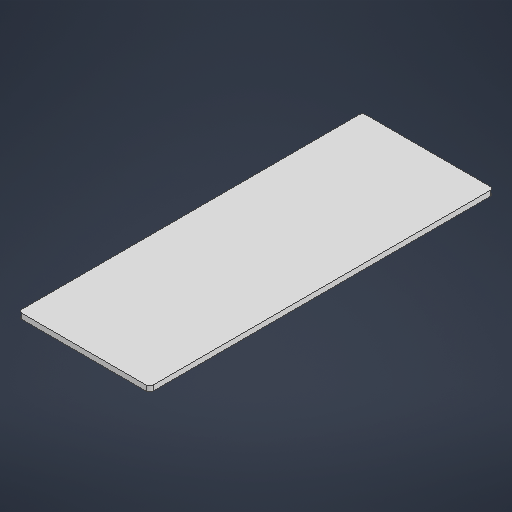
# Autodesk Inventor part: module-lid_command
Saved by Autodesk Inventor 2025.2 (Build 292293000, 293)
## iProperties
Created: 2025-09-05
Part Number: module-lid_command
Material: Generic
Document SubType Name: Modeling
Designer: sam
Density: 1 g/cm^3
Appearance: Default
Author: sam
Autodesk Inventor part; units mm, degrees
ref_plane "YZ Plane" through (0, 0, 0) normal (1, 0, 0) x (0, 1, 0)
ref_plane "XZ Plane" through (0, 0, 0) normal (0, 1, 0) x (-1, 0, 0)
ref_plane "XY Plane" through (0, 0, 0) normal (0, 0, 1) x (1, 0, 0)
sketch "Sketch1" plane through (0, 0, 0) normal (0, 1, 0) x (-1, 0, 0)
  line L0 (-37, -97) -> (37, -97)
  line L1 (37, -97) -> (37, 97)
  line L2 (37, 97) -> (-37, 97)
  line L3 (-37, 97) -> (-37, -97)
  line L4 (-37, -97) -> (37, 97) construction
  line L5 (37, -97) -> (-37, 97) construction
  point P0 (0, 0)
  dimension "d0" = 74
  dimension "d1" = 194
  constraints: 12 end point, 2 midpoint, 2 parallel, 1 horizontal, 1 perpendicular
  measures "d0" distance of L2.end L1.end
  measures "d1" distance of L1.end L0.end
extrude "Extrusion1" add sketch "Sketch1" against normal blind 3
sketch "Sketch2" plane through (0, -3, 0) normal (0, -1, 0) x (1, 0, 0)
  line L0 (-37, 97) -> (-37, -97) projected
  line L1 (-37, -97) -> (37, -97) projected
  line L2 (37, -97) -> (37, 97) projected
  line L3 (37, 97) -> (-37, 97) projected
  line L4 (34, 94) -> (-34, 94)
  line L5 (-34, 94) -> (-34, -94)
  line L6 (-34, -94) -> (34, -94)
  line L7 (34, -94) -> (34, 94)
  line L8 (34, 94) -> (-34, -94) construction
  line L9 (-34, 94) -> (34, -94) construction
  point P0 (0, 0)
  dimension "d4" = 3
  dimension "d5" = 3
  constraints: 12 end point, 2 midpoint, 2 parallel, 1 horizontal, 1 perpendicular
  measures "d4" distance between parallel lines of L5 L0
  measures "d5" distance between parallel lines of L1 L6
extrude "Extrusion2" add sketch "Sketch2" along normal blind 3 contours L7 L6 L5 L4
fillet "Fillet1" radius 2 8 edges at (34, -4.5, 94) (-34, -4.5, 94) (37, -1.5, 97) (-37, -1.5, 97) (34, -4.5, -94) (37, -1.5, -97) (-34, -4.5, -94) (-37, -1.5, -97)
fillet "Fillet2" radius 0.5 8 edges at (-33.4142, -6, 93.4142) (-34, -6, 0) (-33.4142, -6, -93.4142) (0, -6, -94) (33.4142, -6, -93.4142) (34, -6, 0) (33.4142, -6, 93.4142) (0, -6, 94)
body "Solid1"
